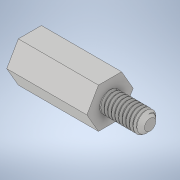
# Autodesk Inventor part: Gewinde
Saved by Autodesk Inventor 2021 (Build 250183000, 183)
## iProperties
Created: 2018-02-01
Part Number: Gewinde
Material: Allgemein
Document SubType Name: Modeling
Designer: Andy
Density: 1 g/cm^3
Appearance: Vorgabe
Author: Andy
## iProperties of the stored document _3D-Druck.ipt
Created: 2021-06-05
Part Number: _3D-Druck
Material: Generisch
Document SubType Name: Modeling
Designer: User
Density: 1 g/cm^3
Appearance: Vorgabe
Author: User
Autodesk Inventor part; units mm, degrees
ref_plane "YZ Plane" through (0, 0, 0) normal (1, 0, 0) x (0, 1, 0)
ref_plane "XZ Plane" through (0, 0, 0) normal (0, 1, 0) x (-1, 0, 0)
ref_plane "XY Plane" through (0, 0, 0) normal (0, 0, 1) x (1, 0, 0)
sketch "Sketch3" plane through (0, 0, 0) normal (0, 0, 1) x (1, 0, 0)
  line L0 (0, 0) -> (15.421869, 0)
  line L1 (0, 2.9) -> (10, 2.9)
  line L2 (10, 2.9) -> (10, 0)
  line L3 (10, 0) -> (0, 0)
  line L4 (10, 1.3) -> (15, 1.3)
  line L5 (15, 1.3) -> (15, 0)
  line L6 (15, 0) -> (10, 0)
  line L7 (10, 0) -> (10, 1.3)
  line L8 (15, 1.3) -> (15.140634, 1.056415)
  arc A0 (15.140634, 1.056415) -> (15.253105, 1.056415) centre (15.196869, 1.088882) ccw
  line L9 (15.253105, 1.056415) -> (15.393738, 1.3)
  line L10 (15, 1.3) -> (14.971869, 1.3)
  line L11 (15.393738, 1.3) -> (15.421869, 1.3)
  line L12 (15, 1.3) -> (15.393738, 1.3)
  line L13 (15.196869, 1.3) -> (15.196869, 1.023947) construction
  line L14 (14.971869, 1.3) -> (15.196869, 1.023947) construction
  line L15 (15.196869, 1.023947) -> (15.421869, 1.3) construction
  line L16 (15.421869, 0) -> (15.421869, 1.3) construction
  line L17 (-0.393745, 1.256438) -> (-0.253124, 1.5)
  line L18 (-0.253124, 1.5) -> (-0.196876, 1.5)
  line L19 (-0.196876, 1.5) -> (-0.056255, 1.256438)
  line L20 (-0.056255, 1.256438) -> (0, 1.256438)
  line L21 (0.056255, 1.256438) -> (0.056255, 1.548713) construction
  line L22 (0.056255, 1.548713) -> (-0.506255, 1.548713) construction
  line L23 (-0.506255, 1.548713) -> (-0.506255, 1.256438) construction
  line L24 (-0.506255, 1.256438) -> (-0.506255, 1.256438) construction
  line L25 (-0.506255, 1.256438) -> (-0.45, 1.256438) construction
  line L26 (-0.45, 1.256438) -> (-0.393745, 1.256438)
  line L27 (0, 1.256438) -> (0.056255, 1.256438) construction
  line L28 (-0.393745, 1.256438) -> (-0.056255, 1.256438) construction
  line L29 (-0.253124, 1.5) -> (-0.225, 1.548713) construction
  line L30 (-0.196876, 1.5) -> (-0.225, 1.548713) construction
  line L31 (-0.506255, 0) -> (0.056255, 0) construction
  line L32 (-0.506255, 1.256438) -> (-0.45, 1.159001) construction
  line L33 (-0.45, 1.159001) -> (-0.393745, 1.256438) construction
  line L34 (-0.056255, 1.256438) -> (0, 1.159001) construction
  line L35 (0, 1.159001) -> (0.056255, 1.256438) construction
  line L36 (-0.225, 1.256438) -> (-0.225, 1.548713) construction
  line L37 (-0.45, 1.159001) -> (0, 1.159001) construction
  line L38 (-0.506255, 0) -> (-0.506255, 1.256438) construction
  line L39 (0.056255, 0) -> (0.056255, 1.256438) construction
  line L40 (10, 1.256437) -> (0, 1.256437)
  line L41 (7, 0) -> (7, 1.256437)
  line L42 (0, 0) -> (0, 2.9)
  line L43 (0, -0.58) -> (0, 3.48)
  line L44 (-0.056255, 1.256438) -> (-0.393745, 1.256438)
  line L45 (15.253105, 1.056415) -> (15.196869, 0.959012)
  line L46 (15.196869, 0.959012) -> (15.140634, 1.056415)
  point P0 (0.524985, 1.771125)
  point P1 (0, 1.256438)
  point P2 (7, 0)
  point P3 (10, 0)
  dimension "d33" = 5.8
  dimension "d36" = 2.6
  dimension "d37" = 5
  dimension "d53" = 60
  dimension "d54" = 0.45
  dimension "d55" = 0.06494
  dimension "d60" = 2.6
  dimension "d61" = 90
  dimension "d62" = 2.0479
  dimension "d63" = 0.02813
  dimension "d64" = -0.02813
  dimension "d80" = 60
  dimension "d81" = 3
  dimension "d82" = 0.45
  dimension "d83" = 2.51288
  dimension "d84" = 0.24356
  dimension "d85" = 0.04871
  dimension "d91" = 2.51288
  dimension "d93" = 3
  dimension "d94" = 90
  dimension "d97" = 10
  dimension "d99" = 0
  constraints: 93 end point, 17 collinear, 9 perpendicular, 9 point on line, 7 parallel, 4 midpoint, 3 point on circle, 2 tangent, 1 centre point, 1 coincident, 7 other
  measures "d33" diameter of L1 L0
  measures "d36" diameter of L4 L0
  measures "d37" distance between parallel lines of L2 L5
  measures "d53" angle of L9 L8
  measures "d54" distance of L10.end L11.end
  measures "d55" radius of A0
  measures "d60" diameter of L11.end L0
  measures "d61" angle of L16 L0
  measures "d62" diameter of L13.end L0
  measures "d63" distance of L10.start L10.end
  measures "d64" distance from line of L10.end L5
  measures "d80" angle of L17 L19
  measures "d81" diameter of L17.end L31
  measures "d82" distance of L25.end L20.end
  measures "d83" diameter of L25.end L31
  measures "d84" distance between parallel lines of L18 L28
  measures "d85" distance from line of L36.end L18
  measures "d91" diameter of L40 L0
  measures "d93" distance between parallel lines of L41 L2
  measures "d94" angle of L43 L3
  measures "d97" distance of L1.start L1.end
  measures "d99" distance from line of L20.end L43
revolve "Revolution1" add sketch "Sketch3" angle 360 about axis through (0, 0, 0) along (1, 0, 0) contours L41 L40 L2 L0 | L42 L1 L2 L40 | L2 L4 L5 L0
chamfer "Fase3" distance 0.6 angle 45 1 edges at (15, -1.3, 0)
coil "Coil2" sketch "Sketch3" operation cut axis through (-10, 0, 0) along (-1, 0, 0) pitch 0.45 turns 11.111111 hand right contours L12 L9 A0 L8 | A0 L45 L46
chamfer "Fase4" distance 0.4 angle 45 1 edges at (0, -1.2564, 0)
coil "Spirale3" sketch "Sketch3" operation cut axis through (0, 0, 0) along (1, 0, 0) pitch 0.45 turns 15.555556 hand right contours L17 L18 L19 L44
sketch "Skizze4" plane through (0, 0, 0) normal (-1, 0, 0) x (0, 0, 1)
  line L0 (-1.443376, 2.5) -> (1.443376, 2.5)
  line L1 (-1.443376, -2.5) -> (1.443376, -2.5)
  line L2 (1.443376, -2.5) -> (2.886751, 0)
  line L3 (2.886751, 0) -> (1.443376, 2.5)
  line L4 (-1.443376, 2.5) -> (-2.886751, 0)
  line L5 (-2.886751, 0) -> (-1.443376, -2.5)
  line L6 (2.886751, 0) -> (-2.886751, 0) construction
  line L7 (0, -2.5) -> (0, 2.5) construction
  circle A0 centre (0, 0) radius 2.9
  dimension "d111" = 5
  dimension "d112" = 5
  constraints: 16 end point, 5 equal length, 3 midpoint, 1 coincident, 1 horizontal, 1 parallel, 1 perpendicular
  measures "d111" distance between parallel lines of L1 L0
  measures "d112" distance between parallel lines of L2 L4
extrude "Extrusion2" cut sketch "Skizze4" against normal through all
equation "\"WINKEL\" = 60deg"
equation "\"D\" = 2.6"
equation "\"P\" = 0.45"
equation "\"D2\" = D - 0.6495 * P"
equation "\"d3\" = 2.0479"
equation "\"D1\" = D - 1.0825 * P"
equation "\"h3\" = 0.6134 * P"
equation "\"H1\" = 0.5413 * P"
equation "\"R\" = 0.1443 * P"
equation "\"H0\" = 0.3897"
equation "\"SW\" = 5"
equation "\"L\" = 5"
equation "\"k\" = 1.7"
equation "\"dw\" = 4.1"
equation "\"b\" = 6"
equation "\"dw2\" = 0.4"
equation "\"d57\" = 60deg"
equation "\"d58\" = 1"
equation "\"d59\" = 0.1443"
equation "\"d86\" = 60deg"
equation "\"d87\" = 3"
equation "\"d88\" = 0.45"
equation "\"d89\" = 2.51288"
equation "\"d90\" = 0.3897"
equation "\"d113\" = 5"
body "Solid1"
